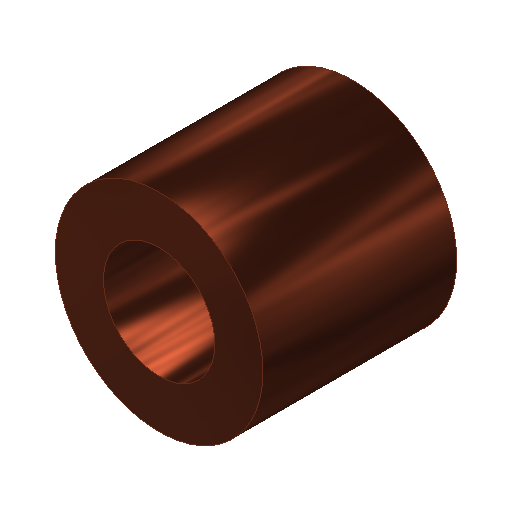
# Autodesk Inventor part: COTS_GENERIC_Solenoid_Actuator_Coil
Saved by Autodesk Inventor 2026.1 (Build 301233000, 233)
## iProperties
Created: 2018-06-14
Part Number: COTS_GENERIC_Solenoid_Actuator_Coil
Material: Generic
Document SubType Name: Modeling
Designer: Andrzej
Density: 1 g/cm^3
Appearance: Copper - Polished
Author: Andrzej
Autodesk Inventor part; units mm, degrees
ref_plane "YZ Plane" through (0, 0, 0) normal (1, 0, 0) x (0, 1, 0)
ref_plane "XZ Plane" through (0, 0, 0) normal (0, 1, 0) x (-1, 0, 0)
ref_plane "XY Plane" through (0, 0, 0) normal (0, 0, 1) x (1, 0, 0)
sketch "Sketch1" plane through (0, 0, 0) normal (0, 0, 1) x (1, 0, 0)
  point P0 (0, 0)
sketch "Sketch2" plane through (0, 0, 0) normal (0, 0, 1) x (1, 0, 0)
  circle A0 centre (0, 0) radius 4.025
  circle A1 centre (0, 0) radius 7.5
  dimension "d0" = 8.05
  dimension "d1" = 15
  constraints: 2 centre point, 2 coincident
  measures "d0" diameter of A0
  measures "d1" diameter of A1
extrude "Extrusion1" add sketch "Sketch2" along normal blind 14
body "Solid1"
